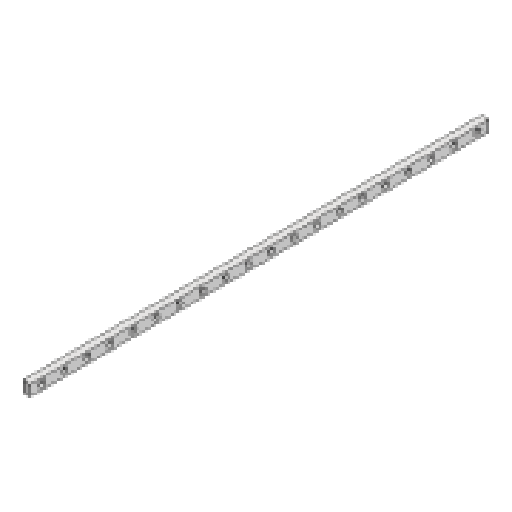
# Autodesk Inventor part: mgn7 300mm rail
Saved by Autodesk Inventor 2023 (Build 270158000, 158)
## iProperties
Created: 2022-10-31
Part Number: mgn7 300mm rail
Material: Generic
Document SubType Name: Modeling
Designer: deli
Density: 1 g/cm^3
Appearance: Default
Author: deli
Autodesk Inventor part; units mm, degrees
ref_plane "YZ Plane" through (0, 0, 0) normal (1, 0, 0) x (0, 1, 0)
ref_plane "XZ Plane" through (0, 0, 0) normal (0, 1, 0) x (-1, 0, 0)
ref_plane "XY Plane" through (0, 0, 0) normal (0, 0, 1) x (1, 0, 0)
sketch "Sketch1" plane through (0, 0, 0) normal (0, 0, 1) x (1, 0, 0)
  line L0 (-12.5153, 6.9424) -> (-7.7153, 6.9424)
  line L1 (-7.7153, 6.9424) -> (-7.7153, -0.0576)
  line L2 (-7.7153, -0.0576) -> (-12.5153, -0.0576)
  line L3 (-12.5153, -0.0576) -> (-12.5153, 6.9424)
  point P0 (0, 0)
  dimension "d0" = 4.8
  dimension "d1" = 7
  constraints: 8 end point, 2 parallel, 1 horizontal, 1 perpendicular
  measures "d0" distance of L0.start L0.end
  measures "d1" distance of L0.end L1.end
extrude "Extrusion1" add sketch "Sketch1" along normal blind 300
sketch "Sketch4" plane through (-7.7153, -0.0576, 0) normal (1, 0, 0) x (0, 0, -1)
  line L0 (0, 0) -> (-300, 0) projected
  line L1 (0, 0) -> (0, 7) projected
  circle A0 centre (-7.5, 3.5) radius 1.2
  circle A1 centre (-22.5, 3.5) radius 1.2
  circle A2 centre (-37.5, 3.5) radius 1.2
  circle A3 centre (-52.5, 3.5) radius 1.2
  circle A4 centre (-67.5, 3.5) radius 1.2
  circle A5 centre (-82.5, 3.5) radius 1.2
  circle A6 centre (-97.5, 3.5) radius 1.2
  circle A7 centre (-112.5, 3.5) radius 1.2
  circle A8 centre (-127.5, 3.5) radius 1.2
  circle A9 centre (-142.5, 3.5) radius 1.2
  circle A10 centre (-157.5, 3.5) radius 1.2
  circle A11 centre (-172.5, 3.5) radius 1.2
  circle A12 centre (-187.5, 3.5) radius 1.2
  circle A13 centre (-202.5, 3.5) radius 1.2
  circle A14 centre (-217.5, 3.5) radius 1.2
  circle A15 centre (-232.5, 3.5) radius 1.2
  circle A16 centre (-247.5, 3.5) radius 1.2
  circle A17 centre (-262.5, 3.5) radius 1.2
  circle A18 centre (-277.5, 3.5) radius 1.2
  circle A19 centre (-292.5, 3.5) radius 1.2
  point P0 (0, 0.0576)
  dimension "d27" = 2.4
  dimension "d28" = 3.5
  dimension "d31" = 15
  dimension "d36" = 285
  dimension "d37" = 7.5
  constraints: 20 centre point, 1 horizontal, 38 other
  measures "d27" diameter of A0
  measures "d28" distance from line of L0 A0.centre
  measures "d31" distance of A0.centre A1.centre
  measures "d36" distance of A19.centre A0.centre
  measures "d37" distance from line of L1 A0.centre
extrude "Extrusion4" cut sketch "Sketch4" against normal blind 10
sketch "Sketch5" plane through (-7.7153, -0.0576, 0) normal (1, 0, 0) x (0, 0, -1)
  circle A0 centre (-7.5, 3.5) radius 1.2 construction
  circle A1 centre (-7.5, 3.5) radius 2.1
  line L0 (0, 0) -> (-300, 0) projected
  circle A2 centre (-22.5, 3.5) radius 2.1
  circle A3 centre (-37.5, 3.5) radius 2.1
  circle A4 centre (-52.5, 3.5) radius 2.1
  circle A5 centre (-67.5, 3.5) radius 2.1
  circle A6 centre (-82.5, 3.5) radius 2.1
  circle A7 centre (-97.5, 3.5) radius 2.1
  circle A8 centre (-112.5, 3.5) radius 2.1
  circle A9 centre (-127.5, 3.5) radius 2.1
  circle A10 centre (-142.5, 3.5) radius 2.1
  circle A11 centre (-157.5, 3.5) radius 2.1
  circle A12 centre (-172.5, 3.5) radius 2.1
  circle A13 centre (-187.5, 3.5) radius 2.1
  circle A14 centre (-202.5, 3.5) radius 2.1
  circle A15 centre (-217.5, 3.5) radius 2.1
  circle A16 centre (-232.5, 3.5) radius 2.1
  circle A17 centre (-247.5, 3.5) radius 2.1
  circle A18 centre (-262.5, 3.5) radius 2.1
  circle A19 centre (-277.5, 3.5) radius 2.1
  circle A20 centre (-292.5, 3.5) radius 2.1
  point P0 (0, 0.0576)
  dimension "d40" = 4.2
  dimension "d43" = 15
  constraints: 20 centre point, 1 coincident, 1 horizontal, 38 other
  measures "d40" diameter of A1
  measures "d43" distance of A1.centre A2.centre
extrude "Extrusion5" cut sketch "Sketch5" against normal blind 2.3
body "Solid1"
